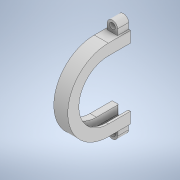
# Autodesk Inventor part: motor_chain_guide
Saved by Autodesk Inventor 2021 (Build 250183000, 183)
## iProperties
Created: 2021-03-18
Part Number: motor_chain_guide
Material: Generic
Document SubType Name: Modeling
Designer: Mateusz
Density: 1 g/cm^3
Appearance: Default
Author: Mateusz
Autodesk Inventor part; units mm, degrees
ref_plane "YZ Plane" through (0, 0, 0) normal (1, 0, 0) x (0, 1, 0)
ref_plane "XZ Plane" through (0, 0, 0) normal (0, 1, 0) x (-1, 0, 0)
ref_plane "XY Plane" through (0, 0, 0) normal (0, 0, 1) x (1, 0, 0)
sketch "Sketch1" plane through (0, 0, 0) normal (1, 0, 0) x (0, 1, 0)
  arc A0 (52, 0) -> (-52, 0) centre (0, 0) ccw
  arc A1 (50.5, 0) -> (-50.5, 0) centre (0, 0) ccw
  arc A2 (55, 0) -> (-55, 0) centre (0, 0) ccw
  line L0 (55, 0) -> (50.5, 0)
  line L1 (-50.5, 0) -> (-55, 0)
  constraints: 6 point on circle, 4 end point, 3 centre point, 1 coincident, 1 horizontal
sketch "Sketch1 outline for Extrusion1" plane through (0, 0, 0) normal (1, 0, 0) x (0, 1, 0)
  arc A0 (-50.5, 0) -> (50.5, 0) centre (0, 0) cw
  line L0 (-52, 0) -> (-50.5, 0)
  arc A1 (52, 0) -> (-52, 0) centre (0, 0) ccw
  line L1 (50.5, 0) -> (52, 0)
extrude "Extrusion1" add sketch "Sketch1 outline for Extrusion1" along normal blind 1.75
sketch "Sketch1 outline for Extrusion4" plane through (0, 0, 0) normal (1, 0, 0) x (0, 1, 0)
  arc A0 (-50.5, 0) -> (50.5, 0) centre (0, 0) cw
  line L0 (-52, 0) -> (-50.5, 0)
  arc A1 (52, 0) -> (-52, 0) centre (0, 0) ccw
  line L1 (50.5, 0) -> (52, 0)
extrude "Extrusion4" add sketch "Sketch1 outline for Extrusion4" against normal blind 1.75
sketch "Sketch1 outline for Extrusion5" plane through (0, 0, 0) normal (1, 0, 0) x (0, 1, 0)
  arc A0 (55, 0) -> (-55, 0) centre (0, 0) ccw
  line L0 (52, 0) -> (55, 0)
  arc A1 (-52, 0) -> (52, 0) centre (0, 0) cw
  line L1 (-55, 0) -> (-52, 0)
extrude "Extrusion5" add sketch "Sketch1 outline for Extrusion5" along normal blind 6.5
sketch "Sketch1 outline for Extrusion6" plane through (0, 0, 0) normal (1, 0, 0) x (0, 1, 0)
  arc A0 (55, 0) -> (-55, 0) centre (0, 0) ccw
  line L0 (52, 0) -> (55, 0)
  arc A1 (-52, 0) -> (52, 0) centre (0, 0) cw
  line L1 (-55, 0) -> (-52, 0)
extrude "Extrusion6" add sketch "Sketch1 outline for Extrusion6" against normal blind 6.5
sketch "Sketch2" plane through (-6.5, 0, 0) normal (-1, 0, 0) x (0, 0, 1)
  arc A0 (0, -55) -> (0, 55) centre (0, 0) ccw
  line L0 (0, -55) -> (0, 55)
  constraints: 2 end point, 2 point on circle, 1 centre point, 1 coincident, 1 vertical
sketch "Sketch2 outline for Extrusion7" plane through (-6.5, 0, 0) normal (-1, 0, 0) x (0, 0, 1)
  arc A0 (0, -55) -> (0, 55) centre (0, 0) ccw
  line L0 (0, 55) -> (0, -55)
extrude "Extrusion7" add sketch "Sketch2 outline for Extrusion7" along normal blind 3
sketch "Sketch3" plane through (1.75, -50.5, 0) normal (0, 0, -1) x (-1, 0, 0)
  line L0 (3.5, 0) -> (0, 0) projected
  line L1 (0, -1.5) -> (0, 0) projected
  line L2 (0, -1.5) -> (-4.75, -1.5) projected
  line L3 (-4.75, -4.5) -> (-4.75, -1.5) projected
  line L4 (-4.75, -4.5) -> (11.25, -4.5) projected
  line L5 (11.25, 105.5) -> (11.25, -4.5) projected
  line L6 (11.25, 105.5) -> (-4.75, 105.5) projected
  line L7 (-4.75, 102.5) -> (-4.75, 105.5) projected
  line L8 (0, 102.5) -> (-4.75, 102.5) projected
  line L9 (0, 101) -> (0, 102.5) projected
  line L10 (0, 101) -> (3.5, 101) projected
  line L11 (3.5, 102.5) -> (3.5, 101) projected
  line L12 (3.5, 102.5) -> (8.25, 102.5) projected
  line L13 (8.25, 102.5) -> (8.25, -1.5) projected
  line L14 (3.5, -1.5) -> (8.25, -1.5) projected
  line L15 (3.5, 0) -> (3.5, -1.5) projected
  point P0 (1.75, 50.5)
sketch "Sketch3 outline for Extrusion8" plane through (1.75, -50.5, 0) normal (0, 0, -1) x (-1, 0, 0)
  line L0 (3.5, -1.5) -> (3.5, 0)
  line L1 (8.25, -1.5) -> (3.5, -1.5)
  line L2 (8.25, 102.5) -> (8.25, -1.5)
  line L3 (3.5, 102.5) -> (8.25, 102.5)
  line L4 (3.5, 101) -> (3.5, 102.5)
  line L5 (0, 101) -> (3.5, 101)
  line L6 (0, 102.5) -> (0, 101)
  line L7 (-4.75, 102.5) -> (0, 102.5)
  line L8 (-4.75, 105.5) -> (-4.75, 102.5)
  line L9 (11.25, 105.5) -> (-4.75, 105.5)
  line L10 (11.25, -4.5) -> (11.25, 105.5)
  line L11 (-4.75, -4.5) -> (11.25, -4.5)
  line L12 (-4.75, -1.5) -> (-4.75, -4.5)
  line L13 (0, -1.5) -> (-4.75, -1.5)
  line L14 (0, 0) -> (0, -1.5)
  line L15 (3.5, 0) -> (0, 0)
extrude "Extrusion8" add sketch "Sketch3 outline for Extrusion8" along normal blind 30
sketch "Sketch4" plane through (-6.5, 0, 0) normal (1, 0, 0) x (0, 0, -1)
  line L0 (0, 35) -> (30, 35)
  line L1 (30, 52) -> (30, -52) projected
  line L2 (0, -35) -> (30, -35)
  arc A0 (0, 35) -> (0, -35) centre (0, 0) ccw
  constraints: 4 end point, 2 point on circle, 2 point on line, 1 centre point, 1 coincident, 1 horizontal, 1 parallel, 1 tangent
sketch "Sketch4 outline for Extrusion9" plane through (-6.5, 0, 0) normal (1, 0, 0) x (0, 0, -1)
  arc A0 (0, 35) -> (0, -35) centre (0, 0) ccw
  line L0 (30, 35) -> (0, 35)
  line L1 (30, -35) -> (30, 35)
  line L2 (0, -35) -> (30, -35)
extrude "Extrusion9" cut sketch "Sketch4 outline for Extrusion9" against normal blind 30
sketch "Sketch6" plane through (6.5, 0, 0) normal (1, 0, 0) x (0, 0, -1)
  arc A0 (0, 52) -> (0, -52) centre (0, 0) ccw projected
  line L0 (0, 52) -> (30, 52) projected
  line L1 (30, 55) -> (30, 52) projected
  line L2 (0, 55) -> (30, 55) projected
  arc A1 (0, 55) -> (0, -55) centre (0, 0) ccw projected
  line L3 (0, -55) -> (30, -55) projected
  line L4 (30, -52) -> (30, -55) projected
  line L5 (0, -52) -> (30, -52) projected
sketch "Sketch6 outline for Extrusion10" plane through (6.5, 0, 0) normal (1, 0, 0) x (0, 0, -1)
  arc A0 (0, 55) -> (0, -55) centre (0, 0) ccw
  line L0 (30, 55) -> (0, 55)
  line L1 (30, 52) -> (30, 55)
  line L2 (0, 52) -> (30, 52)
  arc A1 (0, -52) -> (0, 52) centre (0, 0) cw
  line L3 (30, -52) -> (0, -52)
  line L4 (30, -55) -> (30, -52)
  line L5 (0, -55) -> (30, -55)
extrude "Extrusion10" add sketch "Sketch6 outline for Extrusion10" along normal blind 3
sketch "Sketch7" plane through (1.75, -50.5, -30) normal (0, 0, -1) x (-1, 0, 0)
  line L0 (11.25, 105.5) -> (-7.75, 105.5)
  line L1 (1.75, 109.5) -> (1.75, 113.5)
  circle A0 centre (1.75, 113.5) radius 4
  arc A1 (8.75, 113.5) -> (-5.25, 113.5) centre (1.75, 113.5) ccw
  line L2 (-5.25, 113.5) -> (-5.25, 109.5)
  line L3 (8.75, 113.5) -> (8.75, 109.5)
  line L4 (11.25, -4.5) -> (-7.75, -4.5)
  line L5 (1.75, -8.512708) -> (1.75, -12.512708)
  circle A2 centre (1.75, -12.512708) radius 4
  arc A3 (-5.25, -12.512708) -> (8.75, -12.512708) centre (1.75, -12.512708) ccw
  line L6 (-5.25, -12.512708) -> (-5.25, -8.512708)
  line L7 (0, -1.5) -> (-7.75, -1.5)
  line L8 (8.75, -12.512708) -> (8.75, -8.512708)
  line L9 (-5.25, 109.5) -> (-5.25, 105.5)
  line L10 (8.75, 109.5) -> (8.75, 105.5)
  line L11 (-5.25, -8.512708) -> (-5.25, -4.5)
  line L12 (-7.75, -4.5) -> (11.25, -4.5)
  line L13 (8.75, -8.512708) -> (8.75, -4.5)
  point P0 (1.75, 50.5)
  dimension "d30" = 4
  dimension "d31" = 14
  dimension "d32" = 4
  dimension "d33" = 14
  constraints: 20 end point, 4 coincident, 4 perpendicular, 4 point on circle, 4 point on line, 4 vertical, 2 centre point, 2 parallel, 2 tangent, 2 vertical alignment, 4 other
  measures "d30" distance of L1.start L1.end
  measures "d31" diameter of A1
  measures "d32" distance of L5.start L5.end
  measures "d33" diameter of A3
sketch "Sketch7 outline for Extrusion11" plane through (1.75, -50.5, -30) normal (0, 0, -1) x (-1, 0, 0)
  line L0 (8.75, -12.512708) -> (8.75, -4.5)
  line L1 (8.75, -4.5) -> (-5.25, -4.5)
  line L2 (-5.25, -4.5) -> (-5.25, -12.512708)
  arc A0 (-5.25, -12.512708) -> (8.75, -12.512708) centre (1.75, -12.512708) ccw
  circle A1 centre (1.75, -12.512708) radius 4
  line L3 (-5.25, 113.5) -> (-5.25, 105.5)
  line L4 (-5.25, 105.5) -> (8.75, 105.5)
  line L5 (8.75, 105.5) -> (8.75, 113.5)
  arc A2 (8.75, 113.5) -> (-5.25, 113.5) centre (1.75, 113.5) ccw
  circle A3 centre (1.75, 113.5) radius 4
extrude "Extrusion11" add sketch "Sketch7 outline for Extrusion11" against normal blind 15
fillet "Fillet2" radius 1 21 edges at (-4.125, -52, -30) (-1.75, -51.25, -30) (0, -50.5, -30) (1.75, -51.25, -30) (5.625, -52, -30) (-6.5, 0, 52) (-6.5, 52, -15) (-6.5, -52, -15) (-6.5, -43.5, -30) (-6.5, 43.5, -30) (-4.125, 52, -30) (-1.75, 51.25, -30) (0, 50.5, -30) (1.75, 51.25, -30) (5.625, 52, -30) (1.75, 0, 50.5) (1.75, 50.5, -15) (1.75, -50.5, -15) (-1.75, 0, 50.5) (-1.75, 50.5, -15) (-1.75, -50.5, -15)
sketch "Sketch8" plane through (9.5, 0, 0) normal (1, 0, 0) x (0, 0, -1)
  circle A0 centre (0, 59) radius 1.45
  line L0 (5.45, 59) -> (5.45, 62.763823)
  line L1 (5.45, 59) -> (5.45, 55)
  line L2 (30, 55) -> (0, 55)
  line L3 (0, 63) -> (5.45, 63)
  line L4 (5.45, 63) -> (5.45, 62.763823)
  arc A1 (0, 55) -> (0, -55) centre (0, 0) ccw
  arc A2 (0, 63) -> (-63, 0) centre (0, 0) ccw
  circle A3 centre (-5.443833, 58.748316) radius 1.45
  circle A4 centre (-10.841222, 57.995413) radius 1.45
  circle A5 centre (-16.146116, 56.747713) radius 1.45
  circle A6 centre (-21.313258, 55.015862) radius 1.45
  circle A7 centre (-26.298563, 52.814634) radius 1.45
  circle A8 centre (-31.059498, 50.162811) radius 1.45
  circle A9 centre (-35.555444, 47.083016) radius 1.45
  circle A10 centre (-39.748043, 43.601526) radius 1.45
  circle A11 centre (-43.601526, 39.748043) radius 1.45
  circle A12 centre (-47.083016, 35.555444) radius 1.45
  circle A13 centre (-50.162811, 31.059498) radius 1.45
  circle A14 centre (-52.814634, 26.298563) radius 1.45
  circle A15 centre (-55.015862, 21.313258) radius 1.45
  circle A16 centre (-56.747713, 16.146116) radius 1.45
  circle A17 centre (-57.995413, 10.841222) radius 1.45
  circle A18 centre (-58.748316, 5.443833) radius 1.45
  circle A19 centre (-59, 0) radius 1.45
  line L5 (0, 0) -> (-8.306707, 0)
  line L6 (30, -55) -> (0, -55)
  arc A20 (0, 55) -> (0, -55) centre (0, 0) ccw
  line L7 (-44.547727, 44.547727) -> (-38.890873, 38.890873)
  line L8 (-44.547727, 44.547727) -> (-36.547727, 44.547727) construction
  point P0 (0, -55)
  dimension "d45" = 90
  dimension "d51" = 45
  constraints: 20 centre point, 16 end point, 6 point on circle, 3 point on line, 3 symmetric about line, 2 horizontal, 2 perpendicular, 1 equal length, 1 tangent, 36 other
  measures "d51" angle of L7 L8
sketch "Sketch8 outline for Extrusion12" plane through (9.5, 0, 0) normal (1, 0, 0) x (0, 0, -1)
  line L0 (5.45, 59) -> (5.45, 62.763823)
  line L1 (5.45, 55) -> (5.45, 59)
  line L2 (5.45, 62.763823) -> (5.45, 63)
  line L3 (0, 55) -> (5.45, 55)
  line L4 (5.45, 63) -> (0, 63)
  arc A0 (-38.890873, 38.890873) -> (0, 55) centre (0, 0) cw
  arc A1 (0, 63) -> (-44.547727, 44.547727) centre (0, 0) ccw
  line L5 (-44.547727, 44.547727) -> (-38.890873, 38.890873)
  circle A2 centre (-39.748043, 43.601526) radius 1.45
  circle A3 centre (-35.555444, 47.083016) radius 1.45
  circle A4 centre (-31.059498, 50.162811) radius 1.45
  circle A5 centre (-26.298563, 52.814634) radius 1.45
  circle A6 centre (-21.313258, 55.015862) radius 1.45
  circle A7 centre (-16.146116, 56.747713) radius 1.45
  circle A8 centre (-10.841222, 57.995413) radius 1.45
  circle A9 centre (-5.443833, 58.748316) radius 1.45
  circle A10 centre (0, 59) radius 1.45
extrude "Extrusion12" add sketch "Sketch8 outline for Extrusion12" against normal blind 5
sketch "Sketch9" plane through (-6.5, 0, 0) normal (1, 0, 0) x (0, 0, -1)
  circle A0 centre (0, 0) radius 40
  line L0 (0, 40) -> (30.370061, 40)
  line L1 (30, 35) -> (30, 51)
  line L2 (30.370061, 40) -> (30.370061, 26.031892)
  line L3 (0, -40) -> (36.514522, -40)
  line L4 (36.514522, -40) -> (40, 0)
  dimension "d52" = 80
  constraints: 8 end point, 4 point on circle, 3 perpendicular, 1 centre point, 1 coincident, 1 tangent
  measures "d52" diameter of A0
sketch "Sketch9 outline for Extrusion13" plane through (-6.5, 0, 0) normal (1, 0, 0) x (0, 0, -1)
  line L0 (30.370061, 26.031892) -> (30.370061, 40)
  arc A0 (40, 0) -> (30.370061, 26.031892) centre (0, 0) ccw
  line L1 (36.514522, -40) -> (40, 0)
  line L2 (0, -40) -> (36.514522, -40)
  arc A1 (0, 40) -> (0, -40) centre (0, 0) ccw
  line L3 (30.370061, 40) -> (0, 40)
extrude "Extrusion13" cut sketch "Sketch9 outline for Extrusion13" against normal blind 5
sketch "Sketch10" plane through (4.5, 0, 0) normal (-1, 0, 0) x (0, 0, 1)
  line L0 (-5.45, 63) -> (-5.45, 55)
  line L1 (0, 55) -> (-5.45, 55)
  arc A0 (38.890873, 38.890873) -> (0, 55) centre (0, 0) ccw
  line L2 (38.890873, 38.890873) -> (44.547727, 44.547727)
  arc A1 (44.547727, 44.547727) -> (0, 63) centre (0, 0) ccw
  line L3 (0, 63) -> (-5.45, 63)
  circle A2 centre (39.748043, 43.601526) radius 1.45
  circle A3 centre (35.555444, 47.083016) radius 1.45
  circle A4 centre (31.059498, 50.162811) radius 1.45
  circle A5 centre (26.298563, 52.814634) radius 1.45
  circle A6 centre (21.313258, 55.015862) radius 1.45
  circle A7 centre (16.146116, 56.747713) radius 1.45
  circle A8 centre (10.841222, 57.995413) radius 1.45
  circle A9 centre (5.443833, 58.748316) radius 1.45
  circle A10 centre (0, 59) radius 1.45
sketch "Sketch10 outline for Extrusion14" plane through (4.5, 0, 0) normal (-1, 0, 0) x (0, 0, 1)
  line L0 (38.890873, 38.890873) -> (44.547727, 44.547727)
  arc A0 (0, 55) -> (38.890873, 38.890873) centre (0, 0) cw
  arc A1 (44.547727, 44.547727) -> (0, 63) centre (0, 0) ccw
  line L1 (-5.45, 55) -> (0, 55)
  line L2 (0, 63) -> (-5.45, 63)
  line L3 (-5.45, 63) -> (-5.45, 55)
  circle A2 centre (39.748043, 43.601526) radius 1.45
  circle A3 centre (35.555444, 47.083016) radius 1.45
  circle A4 centre (31.059498, 50.162811) radius 1.45
  circle A5 centre (0, 59) radius 1.45
  circle A6 centre (5.443833, 58.748316) radius 1.45
  circle A7 centre (10.841222, 57.995413) radius 1.45
  circle A8 centre (16.146116, 56.747713) radius 1.45
  circle A9 centre (26.298563, 52.814634) radius 1.45
  circle A10 centre (21.313258, 55.015862) radius 1.45
extrude "Extrusion14" cut sketch "Sketch10 outline for Extrusion14" against normal up to surface (5 mm away)
sketch "Sketch11" plane through (-9.5, 0, 0) normal (-1, 0, 0) x (0, 0, 1)
  arc A0 (0, -40) -> (0, 40) centre (0, 0) ccw
  arc A1 (0, -41.5) -> (0, 41.5) centre (0, 0) ccw
  line L0 (0, 40) -> (-29, 40) projected
  line L1 (-30, 40) -> (-30, 55) projected
  line L2 (0, 40) -> (-30, 40)
  line L3 (0, 41.5) -> (-30, 41.5)
  line L4 (-29, 40) -> (-30, 40) projected
  line L5 (-30, 40) -> (-30, 41.5)
  line L6 (0, -41.5) -> (-30, -41.5)
  line L7 (-30, -51) -> (-30, -40) projected
  line L8 (-30, -41.5) -> (-30, -40)
  line L9 (0, -40) -> (-30, -40) projected
  line L10 (-30, -40) -> (0, -40)
  dimension "d57" = 83
  constraints: 12 end point, 5 perpendicular, 4 point on circle, 2 centre point, 2 coincident, 2 point on line, 1 collinear
  measures "d57" diameter of A1
sketch "Sketch11 outline for Extrusion15" plane through (-9.5, 0, 0) normal (-1, 0, 0) x (0, 0, 1)
  arc A0 (0, 40) -> (0, -40) centre (0, 0) cw
  line L0 (-29, 40) -> (0, 40)
  line L1 (-30, 40) -> (-29, 40)
  line L2 (-30, 41.5) -> (-30, 40)
  line L3 (0, 41.5) -> (-30, 41.5)
  arc A1 (0, -41.5) -> (0, 41.5) centre (0, 0) ccw
  line L4 (-30, -41.5) -> (0, -41.5)
  line L5 (-30, -40) -> (-30, -41.5)
  line L6 (0, -40) -> (-30, -40)
extrude "Extrusion15" add sketch "Sketch11 outline for Extrusion15" along normal blind 5.75
sketch "Sketch12" plane through (9.5, 0, 0) normal (1, 0, 0) x (0, 0, -1)
  line L0 (30, 55) -> (0, 55) projected
  arc A0 (0, 55) -> (0, -55) centre (0, 0) ccw projected
  line L1 (0, -55) -> (30, -55) projected
  line L2 (30, -55) -> (30, -53) projected
  arc A1 (30, -53) -> (29, -52) centre (29, -53) ccw projected
  line L3 (29, -52) -> (0, -52) projected
  arc A2 (0, 52) -> (0, -52) centre (0, 0) ccw projected
  line L4 (0, 52) -> (29, 52) projected
  arc A3 (29, 52) -> (30, 53) centre (29, 53) ccw projected
  line L5 (30, 53) -> (30, 55) projected
  line L6 (0, 40) -> (29, 40) projected
  line L7 (29, 51) -> (29, 40) projected
  line L8 (0, 51) -> (29, 51) projected
  arc A4 (0, 51) -> (0, -51) centre (0, 0) ccw projected
  line L9 (29, -51) -> (0, -51) projected
  line L10 (29, -40) -> (29, -51) projected
  line L11 (29, -40) -> (0, -40) projected
  arc A5 (0, 40) -> (0, -40) centre (0, 0) ccw projected
  line L12 (29, 51) -> (29, 40) projected
  line L13 (30, 40) -> (30, 51) projected
  line L14 (30, 40) -> (29, 40) projected
  line L15 (30, -51) -> (30, -40) projected
  line L16 (29, -40) -> (30, -40) projected
  line L17 (30, -53) -> (30, -51.5) projected
  arc A6 (30, -51.5) -> (29, -50.5) centre (29, -51.5) ccw projected
  line L18 (30, -53) -> (30, -51) projected
  line L19 (30, 51.5) -> (30, 53) projected
  line L20 (30, 51) -> (30, 53) projected
sketch "Sketch12 outline for Extrusion16" plane through (9.5, 0, 0) normal (1, 0, 0) x (0, 0, -1)
  line L0 (29, 40) -> (30, 40)
  line L1 (0, 40) -> (29, 40)
  arc A0 (0, -40) -> (0, 40) centre (0, 0) cw
  line L2 (29, -40) -> (0, -40)
  line L3 (30, -40) -> (29, -40)
  line L4 (30, -51) -> (30, -40)
  line L5 (30, -51.5) -> (30, -51)
  line L6 (30, -53) -> (30, -51.5)
  arc A1 (29, -52) -> (30, -53) centre (29, -53) cw
  line L7 (0, -52) -> (29, -52)
  arc A2 (0, 52) -> (0, -52) centre (0, 0) ccw
  line L8 (29, 52) -> (0, 52)
  arc A3 (30, 53) -> (29, 52) centre (29, 53) cw
  line L9 (30, 51.5) -> (30, 53)
  line L10 (30, 51) -> (30, 51.5)
  line L11 (30, 40) -> (30, 51)
extrude "Extrusion16" add sketch "Sketch12 outline for Extrusion16" against normal blind 3
fillet "Fillet5" radius 1 2 edges at (6.5, 46.5, -30) (6.5, -46.5, -30)
body "Solid1"
